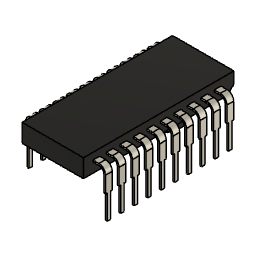
Parameteric_Velocimeter (Autodesk Fusion 360 archive; units mm, degrees)
design "ADNS3080"
Autodesk Fusion 360 part; units mm, degrees
sketch "Sketch1" plane through (0, 0, 0) normal (0, 0, 1) x (1, 0, 0)
  line L0 (-4.55, 6.025) -> (4.55, 6.025)
  line L1 (4.55, 6.025) -> (4.55, -16.275)
  line L2 (4.55, -16.275) -> (-4.55, -16.275)
  line L3 (-4.55, -16.275) -> (-4.55, 6.025)
  line L4 (0, 6.025) -> (0, -16.275) construction
  circle A0 centre (0, 0) radius 0.525
  line L5 (-0.8, 0.8) -> (0.8, 0.8)
  line L6 (0.8, 0.8) -> (0.8, -0.8)
  line L7 (0.8, -0.8) -> (-0.8, -0.8)
  line L8 (-0.8, -0.8) -> (-0.8, 0.8)
  line L9 (0.8, 0.8) -> (-0.8, -0.8) construction
  line L10 (-4.55, -12.88) -> (-6.425, -12.88)
  line L11 (-6.425, -12.88) -> (-6.425, -13.88)
  line L12 (-6.425, -13.88) -> (-4.55, -13.88)
  line L13 (-4.55, -13.88) -> (-4.55, -12.88)
  line L14 (-4.55, -13.38) -> (-6.425, -13.38) construction
  line L15 (-6.425, -11.88) -> (-4.55, -11.88)
  line L16 (-4.55, -11.88) -> (-4.55, -10.88)
  line L17 (-6.425, -10.88) -> (-6.425, -11.88)
  line L18 (-4.55, -10.88) -> (-6.425, -10.88)
  line L19 (-6.425, -9.88) -> (-4.55, -9.88)
  line L20 (-4.55, -9.88) -> (-4.55, -8.88)
  line L21 (-6.425, -8.88) -> (-6.425, -9.88)
  line L22 (-4.55, -8.88) -> (-6.425, -8.88)
  line L23 (-6.425, -7.88) -> (-4.55, -7.88)
  line L24 (-4.55, -7.88) -> (-4.55, -6.88)
  line L25 (-6.425, -6.88) -> (-6.425, -7.88)
  line L26 (-4.55, -6.88) -> (-6.425, -6.88)
  line L27 (-6.425, -5.88) -> (-4.55, -5.88)
  line L28 (-4.55, -5.88) -> (-4.55, -4.88)
  line L29 (-6.425, -4.88) -> (-6.425, -5.88)
  line L30 (-4.55, -4.88) -> (-6.425, -4.88)
  line L31 (-6.425, -3.88) -> (-4.55, -3.88)
  line L32 (-4.55, -3.88) -> (-4.55, -2.88)
  line L33 (-6.425, -2.88) -> (-6.425, -3.88)
  line L34 (-4.55, -2.88) -> (-6.425, -2.88)
  line L35 (-6.425, -1.88) -> (-4.55, -1.88)
  line L36 (-4.55, -1.88) -> (-4.55, -0.88)
  line L37 (-6.425, -0.88) -> (-6.425, -1.88)
  line L38 (-4.55, -0.88) -> (-6.425, -0.88)
  line L39 (-6.425, 0.12) -> (-4.55, 0.12)
  line L40 (-4.55, 0.12) -> (-4.55, 1.12)
  line L41 (-6.425, 1.12) -> (-6.425, 0.12)
  line L42 (-4.55, 1.12) -> (-6.425, 1.12)
  line L43 (-6.425, 2.12) -> (-4.55, 2.12)
  line L44 (-4.55, 2.12) -> (-4.55, 3.12)
  line L45 (-6.425, 3.12) -> (-6.425, 2.12)
  line L46 (-4.55, 3.12) -> (-6.425, 3.12)
  line L47 (-6.425, 4.12) -> (-4.55, 4.12)
  line L48 (-4.55, 4.12) -> (-4.55, 5.12)
  line L49 (-6.425, 5.12) -> (-6.425, 4.12)
  line L50 (-4.55, 5.12) -> (-6.425, 5.12)
  line L51 (4.55, -13.88) -> (6.425, -13.88)
  line L52 (6.425, -13.88) -> (6.425, -14.88)
  line L53 (6.425, -14.88) -> (4.55, -14.88)
  line L54 (4.55, -14.88) -> (4.55, -13.88)
  line L55 (6.425, -14.38) -> (4.55, -14.38) construction
  line L56 (6.425, -12.88) -> (4.55, -12.88)
  line L57 (4.55, -12.88) -> (4.55, -11.88)
  line L58 (6.425, -11.88) -> (6.425, -12.88)
  line L59 (4.55, -11.88) -> (6.425, -11.88)
  line L60 (6.425, -10.88) -> (4.55, -10.88)
  line L61 (4.55, -10.88) -> (4.55, -9.88)
  line L62 (6.425, -9.88) -> (6.425, -10.88)
  line L63 (4.55, -9.88) -> (6.425, -9.88)
  line L64 (6.425, -8.88) -> (4.55, -8.88)
  line L65 (4.55, -8.88) -> (4.55, -7.88)
  line L66 (6.425, -7.88) -> (6.425, -8.88)
  line L67 (4.55, -7.88) -> (6.425, -7.88)
  line L68 (6.425, -6.88) -> (4.55, -6.88)
  line L69 (4.55, -6.88) -> (4.55, -5.88)
  line L70 (6.425, -5.88) -> (6.425, -6.88)
  line L71 (4.55, -5.88) -> (6.425, -5.88)
  line L72 (6.425, -4.88) -> (4.55, -4.88)
  line L73 (4.55, -4.88) -> (4.55, -3.88)
  line L74 (6.425, -3.88) -> (6.425, -4.88)
  line L75 (4.55, -3.88) -> (6.425, -3.88)
  line L76 (6.425, -2.88) -> (4.55, -2.88)
  line L77 (4.55, -2.88) -> (4.55, -1.88)
  line L78 (6.425, -1.88) -> (6.425, -2.88)
  line L79 (4.55, -1.88) -> (6.425, -1.88)
  line L80 (6.425, -0.88) -> (4.55, -0.88)
  line L81 (4.55, -0.88) -> (4.55, 0.12)
  line L82 (6.425, 0.12) -> (6.425, -0.88)
  line L83 (4.55, 0.12) -> (6.425, 0.12)
  line L84 (6.425, 1.12) -> (4.55, 1.12)
  line L85 (4.55, 1.12) -> (4.55, 2.12)
  line L86 (6.425, 2.12) -> (6.425, 1.12)
  line L87 (4.55, 2.12) -> (6.425, 2.12)
  line L88 (6.425, 3.12) -> (4.55, 3.12)
  line L89 (4.55, 3.12) -> (4.55, 4.12)
  line L90 (6.425, 4.12) -> (6.425, 3.12)
  line L91 (4.55, 4.12) -> (6.425, 4.12)
  circle A1 centre (0, 0) radius 2.8
  line L92 (-3.64, 5.025) -> (3.64, 5.025)
  line L93 (3.64, 5.025) -> (3.64, -15.275)
  line L94 (3.64, -15.275) -> (-3.64, -15.275)
  line L95 (-3.64, -15.275) -> (-3.64, 5.025)
  line L96 (-6.425, -13.63) -> (-4.55, -13.63)
  line L97 (-4.55, -13.63) -> (-4.55, -13.13)
  line L98 (-4.55, -13.13) -> (-6.425, -13.13)
  line L99 (-6.425, -13.13) -> (-6.425, -13.63)
  line L100 (4.55, -14.63) -> (6.425, -14.63)
  line L101 (6.425, -14.63) -> (6.425, -14.13)
  line L102 (6.425, -14.13) -> (4.55, -14.13)
  line L103 (4.55, -14.13) -> (4.55, -14.63)
  line L104 (4.55, -12.63) -> (6.425, -12.63)
  line L105 (6.425, -12.63) -> (6.425, -12.13)
  line L106 (4.55, -12.13) -> (4.55, -12.63)
  line L107 (6.425, -12.13) -> (4.55, -12.13)
  line L108 (4.55, -10.63) -> (6.425, -10.63)
  line L109 (6.425, -10.63) -> (6.425, -10.13)
  line L110 (4.55, -10.13) -> (4.55, -10.63)
  line L111 (6.425, -10.13) -> (4.55, -10.13)
  line L112 (4.55, -8.63) -> (6.425, -8.63)
  line L113 (6.425, -8.63) -> (6.425, -8.13)
  line L114 (4.55, -8.13) -> (4.55, -8.63)
  line L115 (6.425, -8.13) -> (4.55, -8.13)
  line L116 (4.55, -6.63) -> (6.425, -6.63)
  line L117 (6.425, -6.63) -> (6.425, -6.13)
  line L118 (4.55, -6.13) -> (4.55, -6.63)
  line L119 (6.425, -6.13) -> (4.55, -6.13)
  line L120 (4.55, -4.63) -> (6.425, -4.63)
  line L121 (6.425, -4.63) -> (6.425, -4.13)
  line L122 (4.55, -4.13) -> (4.55, -4.63)
  line L123 (6.425, -4.13) -> (4.55, -4.13)
  line L124 (4.55, -2.63) -> (6.425, -2.63)
  line L125 (6.425, -2.63) -> (6.425, -2.13)
  line L126 (4.55, -2.13) -> (4.55, -2.63)
  line L127 (6.425, -2.13) -> (4.55, -2.13)
  line L128 (4.55, -0.63) -> (6.425, -0.63)
  line L129 (6.425, -0.63) -> (6.425, -0.13)
  line L130 (4.55, -0.13) -> (4.55, -0.63)
  line L131 (6.425, -0.13) -> (4.55, -0.13)
  line L132 (4.55, 1.37) -> (6.425, 1.37)
  line L133 (6.425, 1.37) -> (6.425, 1.87)
  line L134 (4.55, 1.87) -> (4.55, 1.37)
  line L135 (6.425, 1.87) -> (4.55, 1.87)
  line L136 (4.55, 3.37) -> (6.425, 3.37)
  line L137 (6.425, 3.37) -> (6.425, 3.87)
  line L138 (4.55, 3.87) -> (4.55, 3.37)
  line L139 (6.425, 3.87) -> (4.55, 3.87)
  line L140 (-4.55, -11.13) -> (-6.425, -11.13)
  line L141 (-6.425, -11.13) -> (-6.425, -11.63)
  line L142 (-4.55, -11.63) -> (-4.55, -11.13)
  line L143 (-6.425, -11.63) -> (-4.55, -11.63)
  line L144 (-4.55, -9.13) -> (-6.425, -9.13)
  line L145 (-6.425, -9.13) -> (-6.425, -9.63)
  line L146 (-4.55, -9.63) -> (-4.55, -9.13)
  line L147 (-6.425, -9.63) -> (-4.55, -9.63)
  line L148 (-4.55, -7.13) -> (-6.425, -7.13)
  line L149 (-6.425, -7.13) -> (-6.425, -7.63)
  line L150 (-4.55, -7.63) -> (-4.55, -7.13)
  line L151 (-6.425, -7.63) -> (-4.55, -7.63)
  line L152 (-4.55, -5.13) -> (-6.425, -5.13)
  line L153 (-6.425, -5.13) -> (-6.425, -5.63)
  line L154 (-4.55, -5.63) -> (-4.55, -5.13)
  line L155 (-6.425, -5.63) -> (-4.55, -5.63)
  line L156 (-4.55, -3.13) -> (-6.425, -3.13)
  line L157 (-6.425, -3.13) -> (-6.425, -3.63)
  line L158 (-4.55, -3.63) -> (-4.55, -3.13)
  line L159 (-6.425, -3.63) -> (-4.55, -3.63)
  line L160 (-4.55, -1.13) -> (-6.425, -1.13)
  line L161 (-6.425, -1.13) -> (-6.425, -1.63)
  line L162 (-4.55, -1.63) -> (-4.55, -1.13)
  line L163 (-6.425, -1.63) -> (-4.55, -1.63)
  line L164 (-4.55, 0.87) -> (-6.425, 0.87)
  line L165 (-6.425, 0.87) -> (-6.425, 0.37)
  line L166 (-4.55, 0.37) -> (-4.55, 0.87)
  line L167 (-6.425, 0.37) -> (-4.55, 0.37)
  line L168 (-4.55, 2.87) -> (-6.425, 2.87)
  line L169 (-6.425, 2.87) -> (-6.425, 2.37)
  line L170 (-4.55, 2.37) -> (-4.55, 2.87)
  line L171 (-6.425, 2.37) -> (-4.55, 2.37)
  line L172 (-4.55, 4.87) -> (-6.425, 4.87)
  line L173 (-6.425, 4.87) -> (-6.425, 4.37)
  line L174 (-4.55, 4.37) -> (-4.55, 4.87)
  line L175 (-6.425, 4.37) -> (-4.55, 4.37)
  dimension "d1" = 9.1
  dimension "d2" = 22.3
  dimension "d3" = 6.025
  dimension "d4" = 1.05
  dimension "d5" = 1.6
  dimension "d6" = 1.6
  dimension "d7" = 13.38
  dimension "d8" = 6.425
  dimension "d9" = 1
  dimension "d12" = 0
  dimension "d13" = 2
  dimension "d14" = 1
  dimension "d15" = 1
  dimension "d18" = 0
  dimension "d19" = 2
  dimension "d20" = 5.6
  dimension "d21" = 7.28
  dimension "d22" = 1
  dimension "d23" = 1
  dimension "d31" = 0.5
  dimension "d32" = 0.5
  constraint horizontal L0
  constraint vertical L1
  constraint horizontal L2
  constraint vertical L3
  constraint midpoint L0 L4.start
  constraint midpoint L2 L4.end
  constraint coincident A0.centre L4
  constraint coincident A0.centre A1.centre
  constraint horizontal L5
  constraint vertical L6
  constraint horizontal L7
  constraint vertical L8
  constraint midpoint A0.centre L9
  constraint horizontal L10
  constraint vertical L11
  constraint horizontal L12
  constraint vertical L13
  constraint coincident L3 L10.start
  constraint midpoint L13 L14.start
  constraint midpoint L11 L14.end
  constraint horizontal L51
  constraint vertical L52
  constraint horizontal L53
  constraint vertical L54
  constraint coincident L1 L51.start
  constraint midpoint L52 L55.start
  constraint midpoint L54 L55.end
  constraint concentric A0 A1
  constraint horizontal L92
  constraint vertical L93
  constraint horizontal L94
  constraint vertical L95
  constraint symmetric L4 L93 L95
  constraint horizontal L96
  constraint vertical L97
  constraint horizontal L98
  constraint vertical L99
  constraint coincident L13 L97.end
  constraint coincident L11 L96.start
  constraint symmetric L14 L96 L98
  constraint horizontal L100
  constraint vertical L101
  constraint horizontal L102
  constraint vertical L103
  constraint coincident L52 L101.end
  constraint coincident L1 L100.start
  constraint symmetric L55 L100 L102
  measures "d1" distance of L0.start L0.end
  measures "d2" distance of L0.end L1.end
  measures "d3" distance of A0.centre L0
  measures "d4" diameter of A0
  measures "d5" distance of L5.start L5.end
  measures "d6" distance of L5.start L7.end
  measures "d7" distance of A0.centre L14
  measures "d8" distance of L4 L11
  measures "d9" distance of L10.end L11.end
  measures "d14" distance of L14 L55
  measures "d15" distance of L51.end L52.end
  measures "d20" diameter of A1
  measures "d21" distance of L92.start L92.end
  measures "d22" distance of L0 L92
  measures "d23" distance of L2 L94
  measures "d31" distance of L96 L98
  measures "d32" distance of L100 L102
sketch "Sketch2" plane through (0, 0, 0) normal (0, 1, 0) x (1, 0, 0)
  line L0 (-4.55, -1.71) -> (4.55, -1.71)
  line L1 (4.55, -1.71) -> (4.55, -4.39)
  line L2 (4.55, -4.39) -> (-4.55, -4.39)
  line L3 (-4.55, -4.39) -> (-4.55, -1.71)
  line L4 (-3.64, -1.71) -> (3.64, -1.71)
  line L5 (3.64, -1.71) -> (3.64, -1.21)
  line L6 (3.64, -1.21) -> (-3.64, -1.21)
  line L7 (-3.64, -1.21) -> (-3.64, -1.71)
  line L8 (4.55, -3.4) -> (5.425, -3.4)
  arc A0 (5.425, -3.4) -> (6.425, -2.4) centre (5.425, -2.4) ccw
  line L9 (6.425, -2.4) -> (6.425, 0)
  line L10 (6.425, 0) -> (6.425, 3.65)
  line L11 (4.55, -3.15) -> (5.425, -3.15)
  arc A1 (5.425, -3.15) -> (6.175, -2.4) centre (5.425, -2.4) ccw
  line L12 (6.175, -2.4) -> (6.175, 0)
  line L13 (6.175, 0) -> (6.175, 3.65)
  line L14 (6.425, 0) -> (6.175, 0)
  line L15 (6.425, 3.65) -> (6.175, 3.65)
  line L16 (0, -4.39) -> (0, 0) construction
  line L17 (-4.55, -3.15) -> (-5.425, -3.15)
  line L18 (-6.175, -2.4) -> (-6.175, 0)
  arc A2 (-6.175, -2.4) -> (-5.425, -3.15) centre (-5.425, -2.4) ccw
  line L19 (-4.55, -3.4) -> (-5.425, -3.4)
  line L20 (-6.425, -2.4) -> (-6.425, 0)
  arc A3 (-6.425, -2.4) -> (-5.425, -3.4) centre (-5.425, -2.4) ccw
  line L21 (-6.425, 3.65) -> (-6.175, 3.65)
  line L22 (-6.175, 0) -> (-6.175, 3.65)
  line L23 (-6.425, 0) -> (-6.425, 3.65)
  line L24 (2.8, -1.21) -> (-2.8, -1.21)
  line L25 (-2.8, -1.21) -> (-2.8, 1.04)
  line L26 (-2.8, 1.04) -> (2.8, 1.04)
  line L27 (2.8, 1.04) -> (2.8, -1.21)
  line L28 (3.64, -1.71) -> (3.64, -3.13)
  line L29 (3.64, -3.13) -> (-3.64, -3.13)
  line L30 (-3.64, -3.13) -> (-3.64, -1.71)
  line L31 (0.8, -3.13) -> (-0.8, -3.13)
  line L32 (-0.8, -3.13) -> (-0.8, -2.63)
  line L33 (-0.8, -2.63) -> (0.8, -2.63)
  line L34 (0.8, -2.63) -> (0.8, -3.13)
  line L35 (6.425, -3.4) -> (4.55, -3.4)
  line L36 (4.55, -3.4) -> (4.55, 3.65)
  line L37 (4.55, 3.65) -> (6.425, 3.65)
  line L38 (6.425, 3.65) -> (6.425, -3.4)
  line L39 (-6.425, 3.65) -> (-6.425, -3.4)
  line L40 (-6.425, -3.4) -> (-4.55, -3.4)
  line L41 (-4.55, 3.65) -> (-6.425, 3.65)
  line L42 (-4.55, -3.4) -> (-4.55, 3.65)
  point P0 (-4.55, 0)
  point P1 (4.55, 0)
  point P2 (3.64, 0)
  point P3 (-3.64, 0)
  point P4 (-6.425, 0)
  point P5 (6.425, 0)
  dimension "d24" = 3.18
  dimension "d25" = 1.21
  dimension "d26" = 0.5
  dimension "d27" = 1
  dimension "d28" = 0.99
  dimension "d29" = 7.05
  dimension "d30" = -0.25
  dimension "d37" = 2.25
  dimension "d38" = 5.6
  dimension "d39" = 1.6
  dimension "d40" = 0.5
  dimension "d41" = 3.67
  constraint horizontal L0
  constraint vertical L1
  constraint horizontal L2
  constraint vertical L3
  constraint coincident L3 P0
  constraint coincident L1 P1
  constraint horizontal L4
  constraint vertical L5
  constraint horizontal L6
  constraint vertical L7
  constraint coincident L0 L4.start
  constraint coincident P3 L7
  constraint coincident P2 L5
  constraint coincident L1 L8.start
  constraint perpendicular L1 L8
  constraint tangent L8 A0
  constraint coincident P5 L9.end
  constraint tangent A0 L9
  constraint vertical L9
  constraint parallel L9 L10
  constraint perpendicular L13 L14
  constraint midpoint L2 L16.start
  constraint coincident L16.end origin
  constraint symmetric L8.start L16 L19.start
  constraint symmetric L8.end L16 L19.end
  constraint symmetric A0.end L16 L20.start
  constraint symmetric A0 L16 A3
  constraint symmetric P5 L16 P4
  constraint symmetric L10.end L16 L21.start
  constraint symmetric L11.start L16 L17.start
  constraint symmetric L11.end L16 L17.end
  constraint symmetric A1.end L16 L18.start
  constraint symmetric A1 L16 A2
  constraint symmetric L12.end L16 L18.end
  constraint symmetric L13.end L16 L21.end
  constraint horizontal L24
  constraint vertical L25
  constraint horizontal L26
  constraint vertical L27
  constraint coincident L6 L24.start
  constraint symmetric L16 L25 L27
  constraint perpendicular L4 L28
  constraint perpendicular L16 L29
  constraint perpendicular L0 L30
  constraint horizontal L31
  constraint vertical L32
  constraint horizontal L33
  constraint vertical L34
  constraint coincident L29 L31.start
  constraint symmetric L16 L32 L34
  constraint horizontal L35
  constraint vertical L36
  constraint horizontal L37
  constraint vertical L38
  constraint coincident L13.end L37
  constraint coincident L10 L15.start
  constraint coincident L8.end L35
  constraint symmetric L16 L35.start L39.end
  constraint symmetric L16 L8.start L19.start
  constraint symmetric L16 L36.end L41.start
  constraint symmetric L16 L10.end L21.start
  measures "d24" distance of L2 L6
  measures "d25" distance of L16.end L6
  measures "d26" distance of L4.end L5.end
  measures "d27" radius of A0
  measures "d28" distance of L2 L8
  measures "d29" vertical distance of L8.end L10.end
  measures "d37" distance of L6 L26
  measures "d38" distance of L25.end L26.end
  measures "d39" distance of L32.end L33.end
  measures "d40" distance of L31.end L32.end
  measures "d41" distance of L26 L33
extrude "Extrude1" add sketch "Sketch2" along normal up to surface (6.025 mm away) and the other way up to surface (16.275 mm away) contours L0 L1 L2 L3 L28 L29 L30 L31 L36 L42 | L0 L4 L28 L29 L30 L32 L33 L34 | L29 L31 L32 L33 L34 makes body 1
extrude "Extrude2" cut sketch "Sketch2" along normal up to surface (5.025 mm away) and the other way up to surface (15.275 mm away) contours L0 L4 L28 L29 L30 L32 L33 L34 | L29 L31 L32 L33 L34 bodies 1
extrude "Extrude1'" add sketch "Sketch1" along normal up to surface (0.5 mm away) from surface at 2.63 separate body contours A0 | L5 L6 L7 L8 makes body 2 in component "image sensor"
copy_body "Body->Comp1" bodies 1 removing the originals makes body 3 in component "sensor body"
extrude "Extrude1''" add sketch "Sketch1" along normal up to surface (3.4 mm away) separate body contours L3 L48 L49 L50 L172 | L1 L89 L90 L91 L139 | L3 L48 L49 L172 L173 L174 L175 | L1 L89 L90 L136 L137 L138 L139 | L3 L47 L48 L49 L175 | L1 L88 L89 L90 L136 | L3 L44 L45 L46 L168 | L1 L85 L86 L87 L135 | L3 L44 L45 L168 L169 L170 L171 | L1 L85 L86 L132 L133 L134 L135 | L3 L43 L44 L45 L171 | L1 L84 L85 L86 L132 | L3 L40 L41 L42 L164 | L1 L81 L82 L83 L131 | L3 L40 L41 L164 L165 L166 L167 | L1 L81 L82 L128 L129 L130 L131 | L3 L39 L40 L41 L167 | L1 L80 L81 L82 L128 | L3 L36 L37 L38 L160 | L1 L77 L78 L79 L127 | L3 L36 L37 L160 L161 L162 L163 | L1 L77 L78 L124 L125 L126 L127 | L3 L35 L36 L37 L163 | L1 L76 L77 L78 L124 | L3 L32 L33 L34 L156 | L1 L73 L74 L75 L123 | L3 L32 L33 L156 L157 L158 L159 | L1 L73 L74 L120 L121 L122 L123 | L3 L31 L32 L33 L159 | L1 L72 L73 L74 L120 | L3 L28 L29 L30 L152 | L1 L69 L70 L71 L119 | L3 L28 L29 L152 L153 L154 L155 | L1 L69 L70 L116 L117 L118 L119 | L3 L27 L28 L29 L155 | L1 L68 L69 L70 L116 | L3 L24 L25 L26 L148 | L1 L65 L66 L67 L115 | L3 L24 L25 L148 L149 L150 L151 | L1 L65 L66 L112 L113 L114 L115 | L3 L23 L24 L25 L151 | L1 L64 L65 L66 L112 | L3 L20 L21 L22 L144 | L1 L61 L62 L63 L111 | L3 L20 L21 L144 L145 L146 L147 | L1 L61 L62 L108 L109 L110 L111 | L3 L19 L20 L21 L147 | L1 L60 L61 L62 L108 | L3 L16 L17 L18 L140 | L1 L57 L58 L59 L107 | L3 L16 L17 L140 L141 L142 L143 | L1 L57 L58 L104 L105 L106 L107 | L3 L15 L16 L17 L143 | L1 L56 L57 L58 L104 | L3 L10 L11 L13 L98 | L1 L51 L52 L54 L102 | L3 L11 L13 L96 L97 L98 L99 | L1 L52 L54 L100 L101 L102 L103 | L3 L11 L12 L13 L96 | L1 L52 L53 L54 L100 makes body 4 at (5.8, 0.12, 2.2667) makes body 5 at (5.8, 4.12, 2.2667) makes body 6 at (-5.8, -12.88, 2.2667) makes body 7 at (-5.8, -4.88, 2.2667) makes body 8 at (-5.8, 3.12, 2.2667) makes body 9 at (-5.8, 1.12, 2.2667) makes body 10 at (-5.8, -2.88, 2.2667) makes body 11 at (5.8, -9.88, 2.2667) makes body 12 at (5.8, -5.88, 2.2667) makes body 13 at (5.8, -11.88, 2.2667) makes body 14 at (5.8, -13.88, 2.2667) makes body 15 at (5.8, 2.12, 2.2667) makes body 16 at (-5.8, -10.88, 2.2667) makes body 17 at (-5.8, -0.88, 2.2667) makes body 18 at (-5.8, 5.12, 2.2667) makes body 19 at (-5.8, -6.88, 2.2667) makes body 20 at (-5.8, -8.88, 2.2667) makes body 21 at (5.8, -7.88, 2.2667) makes body 22 at (5.8, -1.88, 2.2667) makes body 23 at (5.8, -3.88, 2.2667) in component "pins"
extrude "Extrude2'" add sketch "Sketch1" against normal up to surface (3.65 mm away) contours L3 L48 L49 L172 L173 L174 L175 | L1 L89 L90 L136 L137 L138 L139 | L3 L44 L45 L168 L169 L170 L171 | L1 L85 L86 L132 L133 L134 L135 | L3 L40 L41 L164 L165 L166 L167 | L1 L81 L82 L128 L129 L130 L131 | L3 L36 L37 L160 L161 L162 L163 | L1 L77 L78 L124 L125 L126 L127 | L3 L32 L33 L156 L157 L158 L159 | L1 L73 L74 L120 L121 L122 L123 | L3 L28 L29 L152 L153 L154 L155 | L1 L69 L70 L116 L117 L118 L119 | L3 L24 L25 L148 L149 L150 L151 | L1 L65 L66 L112 L113 L114 L115 | L3 L20 L21 L144 L145 L146 L147 | L1 L61 L62 L108 L109 L110 L111 | L3 L16 L17 L140 L141 L142 L143 | L1 L57 L58 L104 L105 L106 L107 | L3 L11 L13 L96 L97 L98 L99 | L1 L52 L54 L100 L101 L102 L103 bodies 4 5 6 7 8 9 10 11 12 13 14 15 16 17 18 19 20 21 22 23 in component "pins"
extrude "Extrude3" cut sketch "Sketch2" along normal up to surface (5.12 mm away) and the other way up to surface (14.88 mm away) contours L3 L17 L18 A2 L22 L41 L42 | L1 L11 A1 L12 L13 L36 L37 | A3 L39 L40 | A0 L35 L38 bodies 4 5 6 7 8 9 10 11 12 13 14 15 16 17 18 19 20 21 22 23 in component "pins"
chamfer "Chamfer1" distance 1 angle 45 1 edges at (0, 6.025, 1.71) on bodies 3 in component "sensor body"
extrude "Extrude1'''" add sketch "Sketch1" along normal blind 1 from surface at 1.21 separate body contours L5 L6 L7 L8 | A1 | L92 L93 L94 L95 makes body 24 in component "bottom_cover"
extrude "Extrude2''" add sketch "Sketch1" along normal up to surface (1.21 mm away) and the other way up to surface (1.04 mm away) contours L5 L6 L7 L8 | A1 bodies 24 in component "bottom_cover"
chamfer "Chamfer1'" distance 0.3 angle 45 1 edges at (-2.6105, -1.0125, -1.04) on bodies 24 in component "bottom_cover"
component "image sensor" placed x (1, 0, 0) y (0, 1, 0) z (0, 0, 1) at (0, 0, 0)
component "pins" placed x (1, 0, 0) y (0, 1, 0) z (0, 0, 1) at (0, 0, 0)
component "sensor body" placed x (1, 0, 0) y (0, 1, 0) z (0, 0, 1) at (0, 0, 0)
component "bottom_cover" placed x (1, 0, 0) y (0, 1, 0) z (0, 0, 1) at (0, 0, 0)
equation "d1 = ( 4.55 * 2 ) * 1 mm"
equation "d8 = ( 12.85 / 2 ) * 1 mm"
equation "d15 = d9"
equation "d26 = 3.15 mm - 2.65 mm"
equation "d32 = d31"
